Autodesk Fusion 360 part; units mm, degrees
(part 13 of 18)
  line L7813 (180.127, -19.7823) -> (179.311, -19.7823)
  line L7814 (179.311, -19.5783) -> (180.127, -19.5783)
  line L7815 (180.127, -19.5783) -> (180.127, -19.7823)
  line L7816 (176.8331, -76.9578) -> (177.6491, -76.9578)
  line L7817 (177.6491, -76.9578) -> (177.6491, -76.7538)
  line L7818 (177.6491, -76.7538) -> (176.8331, -76.7538)
  line L7819 (176.8331, -76.7538) -> (176.8331, -76.9578)
  line L7820 (179.821, -77.5359) -> (179.617, -77.5359)
  line L7821 (179.617, -76.1758) -> (179.821, -76.1758)
  line L7822 (179.617, -77.5359) -> (179.617, -76.1758)
  line L7823 (179.821, -76.1758) -> (179.821, -77.5359)
  line L7824 (179.311, -76.9579) -> (179.311, -76.7538)
  line L7825 (179.311, -76.7538) -> (180.127, -76.7538)
  line L7826 (180.127, -76.7538) -> (180.127, -76.9579)
  line L7827 (180.127, -76.9579) -> (179.311, -76.9579)
  line L7828 (176.8331, -57.6911) -> (176.8331, -57.8951)
  line L7829 (176.8331, -57.8951) -> (177.6491, -57.8951)
  line L7830 (177.6491, -57.8951) -> (177.6491, -57.6911)
  line L7831 (177.6491, -57.6911) -> (176.8331, -57.6911)
  line L7832 (179.617, -58.4731) -> (179.617, -57.1131)
  line L7833 (179.821, -57.1131) -> (179.821, -58.4731)
  line L7834 (179.821, -58.4731) -> (179.617, -58.4731)
  line L7835 (179.617, -57.1131) -> (179.821, -57.1131)
  line L7836 (180.127, -57.8951) -> (179.311, -57.8951)
  line L7837 (179.311, -57.6911) -> (180.127, -57.6911)
  line L7838 (180.127, -57.6911) -> (180.127, -57.8951)
  line L7839 (179.311, -57.8951) -> (179.311, -57.6911)
  line L7840 (176.8331, -38.6283) -> (176.8331, -38.8324)
  line L7841 (176.8331, -38.8324) -> (177.6491, -38.8324)
  line L7842 (177.6491, -38.6283) -> (176.8331, -38.6283)
  line L7843 (177.6491, -38.8324) -> (177.6491, -38.6283)
  line L7844 (179.617, -38.0504) -> (179.821, -38.0504)
  line L7845 (179.821, -39.4104) -> (179.617, -39.4104)
  line L7846 (179.821, -38.0504) -> (179.821, -39.4104)
  line L7847 (179.617, -39.4104) -> (179.617, -38.0504)
  line L7848 (179.311, -38.6284) -> (180.127, -38.6284)
  line L7849 (180.127, -38.6284) -> (180.127, -38.8324)
  line L7850 (180.127, -38.8324) -> (179.311, -38.8324)
  line L7851 (179.311, -38.8324) -> (179.311, -38.6284)
  line L7852 (100.6329, -76.7538) -> (100.6329, -76.9578)
  line L7853 (101.4489, -76.7538) -> (100.6329, -76.7538)
  line L7854 (100.6329, -76.9578) -> (101.4489, -76.9578)
  line L7855 (101.4489, -76.9578) -> (101.4489, -76.7538)
  line L7856 (103.4168, -76.1758) -> (103.6208, -76.1758)
  line L7857 (103.6208, -77.5359) -> (103.4168, -77.5359)
  line L7858 (103.6208, -76.1758) -> (103.6208, -77.5359)
  line L7859 (103.4168, -77.5359) -> (103.4168, -76.1758)
  line L7860 (103.9268, -76.9579) -> (103.1108, -76.9579)
  line L7861 (103.1108, -76.7538) -> (103.9268, -76.7538)
  line L7862 (103.9268, -76.7538) -> (103.9268, -76.9579)
  line L7863 (103.1108, -76.9579) -> (103.1108, -76.7538)
  line L7864 (101.4489, -57.6911) -> (100.6329, -57.6911)
  line L7865 (101.4489, -57.8951) -> (101.4489, -57.6911)
  line L7866 (100.6329, -57.6911) -> (100.6329, -57.8951)
  line L7867 (100.6329, -57.8951) -> (101.4489, -57.8951)
  line L7868 (103.4168, -58.4731) -> (103.4168, -57.1131)
  line L7869 (103.4168, -57.1131) -> (103.6208, -57.1131)
  line L7870 (103.6208, -58.4731) -> (103.4168, -58.4731)
  line L7871 (103.6208, -57.1131) -> (103.6208, -58.4731)
  line L7872 (103.9268, -57.8951) -> (103.1108, -57.8951)
  line L7873 (103.9268, -57.6911) -> (103.9268, -57.8951)
  line L7874 (103.1108, -57.6911) -> (103.9268, -57.6911)
  line L7875 (103.1108, -57.8951) -> (103.1108, -57.6911)
  line L7876 (101.4489, -19.5783) -> (100.6329, -19.5783)
  line L7877 (100.6329, -19.5783) -> (100.6329, -19.7823)
  line L7878 (101.4489, -19.7823) -> (101.4489, -19.5783)
  line L7879 (100.6329, -19.7823) -> (101.4489, -19.7823)
  line L7880 (103.6208, -20.3604) -> (103.4168, -20.3604)
  line L7881 (103.6208, -19.0003) -> (103.6208, -20.3604)
  line L7882 (103.4168, -19.0003) -> (103.6208, -19.0003)
  line L7883 (103.4168, -20.3604) -> (103.4168, -19.0003)
  line L7884 (103.1108, -19.7823) -> (103.1108, -19.5783)
  line L7885 (103.9268, -19.7823) -> (103.1108, -19.7823)
  line L7886 (103.9268, -19.5783) -> (103.9268, -19.7823)
  line L7887 (103.1108, -19.5783) -> (103.9268, -19.5783)
  line L7888 (100.6329, -38.8324) -> (101.4489, -38.8324)
  line L7889 (101.4489, -38.6283) -> (100.6329, -38.6283)
  line L7890 (101.4489, -38.8324) -> (101.4489, -38.6283)
  line L7891 (100.6329, -38.6283) -> (100.6329, -38.8324)
  line L7892 (103.4168, -39.4104) -> (103.4168, -38.0504)
  line L7893 (103.6208, -38.0504) -> (103.6208, -39.4104)
  line L7894 (103.6208, -39.4104) -> (103.4168, -39.4104)
  line L7895 (103.4168, -38.0504) -> (103.6208, -38.0504)
  line L7896 (103.1108, -38.8324) -> (103.1108, -38.6284)
  line L7897 (103.9268, -38.8324) -> (103.1108, -38.8324)
  line L7898 (103.9268, -38.6284) -> (103.9268, -38.8324)
  line L7899 (103.1108, -38.6284) -> (103.9268, -38.6284)
  line L7900 (120.499, -19.5783) -> (119.683, -19.5783)
  line L7901 (119.683, -19.5783) -> (119.683, -19.7823)
  line L7902 (120.499, -19.7823) -> (120.499, -19.5783)
  line L7903 (119.683, -19.7823) -> (120.499, -19.7823)
  line L7904 (122.6709, -19.0003) -> (122.6709, -20.3604)
  line L7905 (122.4669, -20.3604) -> (122.4669, -19.0003)
  line L7906 (122.4669, -19.0003) -> (122.6709, -19.0003)
  line L7907 (122.6709, -20.3604) -> (122.4669, -20.3604)
  line L7908 (122.1609, -19.7823) -> (122.1609, -19.5783)
  line L7909 (122.1609, -19.5783) -> (122.9769, -19.5783)
  line L7910 (122.9769, -19.7823) -> (122.1609, -19.7823)
  line L7911 (122.9769, -19.5783) -> (122.9769, -19.7823)
  line L7912 (119.683, -57.8951) -> (120.499, -57.8951)
  line L7913 (120.499, -57.8951) -> (120.499, -57.6911)
  line L7914 (119.683, -57.6911) -> (119.683, -57.8951)
  line L7915 (120.499, -57.6911) -> (119.683, -57.6911)
  line L7916 (122.4669, -57.1131) -> (122.6709, -57.1131)
  line L7917 (122.6709, -57.1131) -> (122.6709, -58.4731)
  line L7918 (122.6709, -58.4731) -> (122.4669, -58.4731)
  line L7919 (122.4669, -58.4731) -> (122.4669, -57.1131)
  line L7920 (122.9769, -57.8951) -> (122.1609, -57.8951)
  line L7921 (122.1609, -57.8951) -> (122.1609, -57.6911)
  line L7922 (122.9769, -57.6911) -> (122.9769, -57.8951)
  line L7923 (122.1609, -57.6911) -> (122.9769, -57.6911)
  line L7924 (119.683, -38.6283) -> (119.683, -38.8324)
  line L7925 (119.683, -38.8324) -> (120.499, -38.8324)
  line L7926 (120.499, -38.6283) -> (119.683, -38.6283)
  line L7927 (120.499, -38.8324) -> (120.499, -38.6283)
  line L7928 (122.6709, -38.0504) -> (122.6709, -39.4104)
  line L7929 (122.6709, -39.4104) -> (122.4669, -39.4104)
  line L7930 (122.4669, -38.0504) -> (122.6709, -38.0504)
  line L7931 (122.4669, -39.4104) -> (122.4669, -38.0504)
  line L7932 (122.9769, -38.8324) -> (122.1609, -38.8324)
  line L7933 (122.1609, -38.6284) -> (122.9769, -38.6284)
  line L7934 (122.1609, -38.8324) -> (122.1609, -38.6284)
  line L7935 (122.9769, -38.6284) -> (122.9769, -38.8324)
  line L7936 (120.499, -76.9578) -> (120.499, -76.7538)
  line L7937 (120.499, -76.7538) -> (119.683, -76.7538)
  line L7938 (119.683, -76.7538) -> (119.683, -76.9578)
  line L7939 (119.683, -76.9578) -> (120.499, -76.9578)
  line L7940 (122.4669, -76.1758) -> (122.6709, -76.1758)
  line L7941 (122.6709, -76.1758) -> (122.6709, -77.5359)
  line L7942 (122.4669, -77.5359) -> (122.4669, -76.1758)
  line L7943 (122.6709, -77.5359) -> (122.4669, -77.5359)
  line L7944 (122.1609, -76.9579) -> (122.1609, -76.7538)
  line L7945 (122.9769, -76.7538) -> (122.9769, -76.9579)
  line L7946 (122.1609, -76.7538) -> (122.9769, -76.7538)
  line L7947 (122.9769, -76.9579) -> (122.1609, -76.9579)
  line L7948 (6.1988, -76.7538) -> (5.3828, -76.7538)
  line L7949 (5.3828, -76.9578) -> (6.1988, -76.9578)
  line L7950 (6.1988, -76.9578) -> (6.1988, -76.7538)
  line L7951 (5.3828, -76.7538) -> (5.3828, -76.9578)
  line L7952 (8.1666, -77.5359) -> (8.1666, -76.1758)
  line L7953 (8.1666, -76.1758) -> (8.3706, -76.1758)
  line L7954 (8.3706, -77.5359) -> (8.1666, -77.5359)
  line L7955 (8.3706, -76.1758) -> (8.3706, -77.5359)
  line L7956 (8.6766, -76.9579) -> (7.8606, -76.9579)
  line L7957 (7.8606, -76.7538) -> (8.6766, -76.7538)
  line L7958 (8.6766, -76.7538) -> (8.6766, -76.9579)
  line L7959 (7.8606, -76.9579) -> (7.8606, -76.7538)
  line L7960 (24.4328, -76.9578) -> (25.2488, -76.9578)
  line L7961 (25.2488, -76.7538) -> (24.4328, -76.7538)
  line L7962 (25.2488, -76.9578) -> (25.2488, -76.7538)
  line L7963 (24.4328, -76.7538) -> (24.4328, -76.9578)
  line L7964 (27.2167, -77.5359) -> (27.2167, -76.1758)
  line L7965 (27.2167, -76.1758) -> (27.4207, -76.1758)
  line L7966 (27.4207, -77.5359) -> (27.2167, -77.5359)
  line L7967 (27.4207, -76.1758) -> (27.4207, -77.5359)
  line L7968 (26.9107, -76.9579) -> (26.9107, -76.7538)
  line L7969 (27.7267, -76.7538) -> (27.7267, -76.9579)
  line L7970 (27.7267, -76.9579) -> (26.9107, -76.9579)
  line L7971 (26.9107, -76.7538) -> (27.7267, -76.7538)
  line L7972 (43.4828, -76.7538) -> (43.4828, -76.9578)
  line L7973 (44.2988, -76.9578) -> (44.2988, -76.7538)
  line L7974 (43.4828, -76.9578) -> (44.2988, -76.9578)
  line L7975 (44.2988, -76.7538) -> (43.4828, -76.7538)
  line L7976 (46.2667, -77.5359) -> (46.2667, -76.1758)
  line L7977 (46.4707, -76.1758) -> (46.4707, -77.5359)
  line L7978 (46.4707, -77.5359) -> (46.2667, -77.5359)
  line L7979 (46.2667, -76.1758) -> (46.4707, -76.1758)
  line L7980 (45.9607, -76.7538) -> (46.7767, -76.7538)
  line L7981 (45.9607, -76.9579) -> (45.9607, -76.7538)
  line L7982 (46.7767, -76.9579) -> (45.9607, -76.9579)
  line L7983 (46.7767, -76.7538) -> (46.7767, -76.9579)
  line L7984 (62.5329, -19.5783) -> (62.5329, -19.7823)
  line L7985 (62.5329, -19.7823) -> (63.3489, -19.7823)
  line L7986 (63.3489, -19.5783) -> (62.5329, -19.5783)
  line L7987 (63.3489, -19.7823) -> (63.3489, -19.5783)
  line L7988 (65.3167, -20.3604) -> (65.3167, -19.0003)
  line L7989 (65.5208, -19.0003) -> (65.5208, -20.3604)
  line L7990 (65.5208, -20.3604) -> (65.3167, -20.3604)
  line L7991 (65.3167, -19.0003) -> (65.5208, -19.0003)
  line L7992 (65.8267, -19.7823) -> (65.0107, -19.7823)
  line L7993 (65.8267, -19.5783) -> (65.8267, -19.7823)
  line L7994 (65.0107, -19.5783) -> (65.8267, -19.5783)
  line L7995 (65.0107, -19.7823) -> (65.0107, -19.5783)
  line L7996 (62.5329, -76.7538) -> (62.5329, -76.9578)
  line L7997 (62.5329, -76.9578) -> (63.3489, -76.9578)
  line L7998 (63.3489, -76.9578) -> (63.3489, -76.7538)
  line L7999 (63.3489, -76.7538) -> (62.5329, -76.7538)
  line L8000 (65.5208, -77.5359) -> (65.3167, -77.5359)
  line L8001 (65.5208, -76.1758) -> (65.5208, -77.5359)
  line L8002 (65.3167, -77.5359) -> (65.3167, -76.1758)
  line L8003 (65.3167, -76.1758) -> (65.5208, -76.1758)
  line L8004 (65.0107, -76.9579) -> (65.0107, -76.7538)
  line L8005 (65.8267, -76.7538) -> (65.8267, -76.9579)
  line L8006 (65.8267, -76.9579) -> (65.0107, -76.9579)
  line L8007 (65.0107, -76.7538) -> (65.8267, -76.7538)
  line L8008 (63.3489, -38.8324) -> (63.3489, -38.6283)
  line L8009 (62.5329, -38.6283) -> (62.5329, -38.8324)
  line L8010 (62.5329, -38.8324) -> (63.3489, -38.8324)
  line L8011 (63.3489, -38.6283) -> (62.5329, -38.6283)
  line L8012 (65.3167, -38.0504) -> (65.5208, -38.0504)
  line L8013 (65.5208, -38.0504) -> (65.5208, -39.4104)
  line L8014 (65.3167, -39.4104) -> (65.3167, -38.0504)
  line L8015 (65.5208, -39.4104) -> (65.3167, -39.4104)
  line L8016 (65.0107, -38.6284) -> (65.8267, -38.6284)
  line L8017 (65.8267, -38.6284) -> (65.8267, -38.8324)
  line L8018 (65.8267, -38.8324) -> (65.0107, -38.8324)
  line L8019 (65.0107, -38.8324) -> (65.0107, -38.6284)
  line L8020 (62.5329, -57.6911) -> (62.5329, -57.8951)
  line L8021 (62.5329, -57.8951) -> (63.3489, -57.8951)
  line L8022 (63.3489, -57.6911) -> (62.5329, -57.6911)
  line L8023 (63.3489, -57.8951) -> (63.3489, -57.6911)
  line L8024 (65.3167, -57.1131) -> (65.5208, -57.1131)
  line L8025 (65.5208, -58.4731) -> (65.3167, -58.4731)
  line L8026 (65.3167, -58.4731) -> (65.3167, -57.1131)
  line L8027 (65.5208, -57.1131) -> (65.5208, -58.4731)
  line L8028 (65.8267, -57.6911) -> (65.8267, -57.8951)
  line L8029 (65.8267, -57.8951) -> (65.0107, -57.8951)
  line L8030 (65.0107, -57.6911) -> (65.8267, -57.6911)
  line L8031 (65.0107, -57.8951) -> (65.0107, -57.6911)
  line L8032 (82.3989, -38.6283) -> (81.5829, -38.6283)
  line L8033 (81.5829, -38.6283) -> (81.5829, -38.8324)
  line L8034 (82.3989, -38.8324) -> (82.3989, -38.6283)
  line L8035 (81.5829, -38.8324) -> (82.3989, -38.8324)
  line L8036 (84.5708, -38.0504) -> (84.5708, -39.4104)
  line L8037 (84.5708, -39.4104) -> (84.3668, -39.4104)
  line L8038 (84.3668, -39.4104) -> (84.3668, -38.0504)
  line L8039 (84.3668, -38.0504) -> (84.5708, -38.0504)
  line L8040 (84.0608, -38.8324) -> (84.0608, -38.6284)
  line L8041 (84.0608, -38.6284) -> (84.8768, -38.6284)
  line L8042 (84.8768, -38.6284) -> (84.8768, -38.8324)
  line L8043 (84.8768, -38.8324) -> (84.0608, -38.8324)
  line L8044 (82.3989, -76.7538) -> (81.5829, -76.7538)
  line L8045 (81.5829, -76.7538) -> (81.5829, -76.9578)
  line L8046 (81.5829, -76.9578) -> (82.3989, -76.9578)
  line L8047 (82.3989, -76.9578) -> (82.3989, -76.7538)
  line L8048 (84.3668, -77.5359) -> (84.3668, -76.1758)
  line L8049 (84.5708, -77.5359) -> (84.3668, -77.5359)
  line L8050 (84.3668, -76.1758) -> (84.5708, -76.1758)
  line L8051 (84.5708, -76.1758) -> (84.5708, -77.5359)
  line L8052 (84.0608, -76.7538) -> (84.8768, -76.7538)
  line L8053 (84.0608, -76.9579) -> (84.0608, -76.7538)
  line L8054 (84.8768, -76.7538) -> (84.8768, -76.9579)
  line L8055 (84.8768, -76.9579) -> (84.0608, -76.9579)
  line L8056 (81.5829, -19.5783) -> (81.5829, -19.7823)
  line L8057 (82.3989, -19.7823) -> (82.3989, -19.5783)
  line L8058 (81.5829, -19.7823) -> (82.3989, -19.7823)
  line L8059 (82.3989, -19.5783) -> (81.5829, -19.5783)
  line L8060 (84.3668, -19.0003) -> (84.5708, -19.0003)
  line L8061 (84.5708, -19.0003) -> (84.5708, -20.3604)
  line L8062 (84.5708, -20.3604) -> (84.3668, -20.3604)
  line L8063 (84.3668, -20.3604) -> (84.3668, -19.0003)
  line L8064 (84.0608, -19.7823) -> (84.0608, -19.5783)
  line L8065 (84.8768, -19.7823) -> (84.0608, -19.7823)
  line L8066 (84.0608, -19.5783) -> (84.8768, -19.5783)
  line L8067 (84.8768, -19.5783) -> (84.8768, -19.7823)
  line L8068 (82.3989, -57.8951) -> (82.3989, -57.6911)
  line L8069 (81.5829, -57.6911) -> (81.5829, -57.8951)
  line L8070 (81.5829, -57.8951) -> (82.3989, -57.8951)
  line L8071 (82.3989, -57.6911) -> (81.5829, -57.6911)
  line L8072 (84.5708, -57.1131) -> (84.5708, -58.4731)
  line L8073 (84.5708, -58.4731) -> (84.3668, -58.4731)
  line L8074 (84.3668, -57.1131) -> (84.5708, -57.1131)
  line L8075 (84.3668, -58.4731) -> (84.3668, -57.1131)
  line L8076 (84.8768, -57.8951) -> (84.0608, -57.8951)
  line L8077 (84.0608, -57.6911) -> (84.8768, -57.6911)
  line L8078 (84.8768, -57.6911) -> (84.8768, -57.8951)
  line L8079 (84.0608, -57.8951) -> (84.0608, -57.6911)
  line L8080 (6.1988, -57.8951) -> (6.1988, -57.6911)
  line L8081 (5.3828, -57.6911) -> (5.3828, -57.8951)
  line L8082 (5.3828, -57.8951) -> (6.1988, -57.8951)
  line L8083 (6.1988, -57.6911) -> (5.3828, -57.6911)
  line L8084 (8.1666, -58.4731) -> (8.1666, -57.1131)
  line L8085 (8.3706, -58.4731) -> (8.1666, -58.4731)
  line L8086 (8.1666, -57.1131) -> (8.3706, -57.1131)
  line L8087 (8.3706, -57.1131) -> (8.3706, -58.4731)
  line L8088 (7.8606, -57.6911) -> (8.6766, -57.6911)
  line L8089 (8.6766, -57.8951) -> (7.8606, -57.8951)
  line L8090 (8.6766, -57.6911) -> (8.6766, -57.8951)
  line L8091 (7.8606, -57.8951) -> (7.8606, -57.6911)
  line L8092 (5.3828, -19.5783) -> (5.3828, -19.7823)
  line L8093 (5.3828, -19.7823) -> (6.1988, -19.7823)
  line L8094 (6.1988, -19.5783) -> (5.3828, -19.5783)
  line L8095 (6.1988, -19.7823) -> (6.1988, -19.5783)
  line L8096 (8.3706, -20.3604) -> (8.1666, -20.3604)
  line L8097 (8.1666, -20.3604) -> (8.1666, -19.0003)
  line L8098 (8.1666, -19.0003) -> (8.3706, -19.0003)
  line L8099 (8.3706, -19.0003) -> (8.3706, -20.3604)
  line L8100 (7.8606, -19.7823) -> (7.8606, -19.5783)
  line L8101 (8.6766, -19.7823) -> (7.8606, -19.7823)
  line L8102 (7.8606, -19.5783) -> (8.6766, -19.5783)
  line L8103 (8.6766, -19.5783) -> (8.6766, -19.7823)
  line L8104 (6.1988, -38.8324) -> (6.1988, -38.6283)
  line L8105 (5.3828, -38.6283) -> (5.3828, -38.8324)
  line L8106 (6.1988, -38.6283) -> (5.3828, -38.6283)
  line L8107 (5.3828, -38.8324) -> (6.1988, -38.8324)
  line L8108 (8.1666, -39.4104) -> (8.1666, -38.0504)
  line L8109 (8.1666, -38.0504) -> (8.3706, -38.0504)
  line L8110 (8.3706, -39.4104) -> (8.1666, -39.4104)
  line L8111 (8.3706, -38.0504) -> (8.3706, -39.4104)
  line L8112 (7.8606, -38.8324) -> (7.8606, -38.6284)
  line L8113 (7.8606, -38.6284) -> (8.6766, -38.6284)
  line L8114 (8.6766, -38.6284) -> (8.6766, -38.8324)
  line L8115 (8.6766, -38.8324) -> (7.8606, -38.8324)
  line L8116 (25.2488, -38.8324) -> (25.2488, -38.6283)
  line L8117 (24.4328, -38.6283) -> (24.4328, -38.8324)
  line L8118 (25.2488, -38.6283) -> (24.4328, -38.6283)
  line L8119 (24.4328, -38.8324) -> (25.2488, -38.8324)
  line L8120 (27.2167, -39.4104) -> (27.2167, -38.0504)
  line L8121 (27.4207, -39.4104) -> (27.2167, -39.4104)
  line L8122 (27.2167, -38.0504) -> (27.4207, -38.0504)
  line L8123 (27.4207, -38.0504) -> (27.4207, -39.4104)
  line L8124 (26.9107, -38.8324) -> (26.9107, -38.6284)
  line L8125 (27.7267, -38.8324) -> (26.9107, -38.8324)
  line L8126 (27.7267, -38.6284) -> (27.7267, -38.8324)
  line L8127 (26.9107, -38.6284) -> (27.7267, -38.6284)
  line L8128 (24.4328, -19.7823) -> (25.2488, -19.7823)
  line L8129 (25.2488, -19.5783) -> (24.4328, -19.5783)
  line L8130 (25.2488, -19.7823) -> (25.2488, -19.5783)
  line L8131 (24.4328, -19.5783) -> (24.4328, -19.7823)
  line L8132 (27.2167, -20.3604) -> (27.2167, -19.0003)
  line L8133 (27.4207, -20.3604) -> (27.2167, -20.3604)
  line L8134 (27.4207, -19.0003) -> (27.4207, -20.3604)
  line L8135 (27.2167, -19.0003) -> (27.4207, -19.0003)
  line L8136 (27.7267, -19.7823) -> (26.9107, -19.7823)
  line L8137 (26.9107, -19.5783) -> (27.7267, -19.5783)
  line L8138 (27.7267, -19.5783) -> (27.7267, -19.7823)
  line L8139 (26.9107, -19.7823) -> (26.9107, -19.5783)
  line L8140 (25.2488, -57.6911) -> (24.4328, -57.6911)
  line L8141 (24.4328, -57.8951) -> (25.2488, -57.8951)
  line L8142 (24.4328, -57.6911) -> (24.4328, -57.8951)
  line L8143 (25.2488, -57.8951) -> (25.2488, -57.6911)
  line L8144 (27.4207, -58.4731) -> (27.2167, -58.4731)
  line L8145 (27.4207, -57.1131) -> (27.4207, -58.4731)
  line L8146 (27.2167, -57.1131) -> (27.4207, -57.1131)
  line L8147 (27.2167, -58.4731) -> (27.2167, -57.1131)
  line L8148 (27.7267, -57.8951) -> (26.9107, -57.8951)
  line L8149 (26.9107, -57.6911) -> (27.7267, -57.6911)
  line L8150 (27.7267, -57.6911) -> (27.7267, -57.8951)
  line L8151 (26.9107, -57.8951) -> (26.9107, -57.6911)
  line L8152 (43.4828, -19.7823) -> (44.2988, -19.7823)
  line L8153 (43.4828, -19.5783) -> (43.4828, -19.7823)
  line L8154 (44.2988, -19.7823) -> (44.2988, -19.5783)
  line L8155 (44.2988, -19.5783) -> (43.4828, -19.5783)
  line L8156 (46.4707, -20.3604) -> (46.2667, -20.3604)
  line L8157 (46.2667, -20.3604) -> (46.2667, -19.0003)
  line L8158 (46.4707, -19.0003) -> (46.4707, -20.3604)
  line L8159 (46.2667, -19.0003) -> (46.4707, -19.0003)
  line L8160 (45.9607, -19.7823) -> (45.9607, -19.5783)
  line L8161 (46.7767, -19.5783) -> (46.7767, -19.7823)
  line L8162 (45.9607, -19.5783) -> (46.7767, -19.5783)
  line L8163 (46.7767, -19.7823) -> (45.9607, -19.7823)
  line L8164 (43.4828, -57.8951) -> (44.2988, -57.8951)
  line L8165 (44.2988, -57.6911) -> (43.4828, -57.6911)
  line L8166 (44.2988, -57.8951) -> (44.2988, -57.6911)
  line L8167 (43.4828, -57.6911) -> (43.4828, -57.8951)
  line L8168 (46.4707, -58.4731) -> (46.2667, -58.4731)
  line L8169 (46.4707, -57.1131) -> (46.4707, -58.4731)
  line L8170 (46.2667, -58.4731) -> (46.2667, -57.1131)
  line L8171 (46.2667, -57.1131) -> (46.4707, -57.1131)
  line L8172 (45.9607, -57.8951) -> (45.9607, -57.6911)
  line L8173 (45.9607, -57.6911) -> (46.7767, -57.6911)
  line L8174 (46.7767, -57.8951) -> (45.9607, -57.8951)
  line L8175 (46.7767, -57.6911) -> (46.7767, -57.8951)
  line L8176 (44.2988, -38.8324) -> (44.2988, -38.6283)
  line L8177 (43.4828, -38.8324) -> (44.2988, -38.8324)
  line L8178 (43.4828, -38.6283) -> (43.4828, -38.8324)
  line L8179 (44.2988, -38.6283) -> (43.4828, -38.6283)
  line L8180 (46.4707, -39.4104) -> (46.2667, -39.4104)
  line L8181 (46.2667, -38.0504) -> (46.4707, -38.0504)
  line L8182 (46.4707, -38.0504) -> (46.4707, -39.4104)
  line L8183 (46.2667, -39.4104) -> (46.2667, -38.0504)
  line L8184 (46.7767, -38.6284) -> (46.7767, -38.8324)
  line L8185 (45.9607, -38.6284) -> (46.7767, -38.6284)
  line L8186 (46.7767, -38.8324) -> (45.9607, -38.8324)
  line L8187 (45.9607, -38.8324) -> (45.9607, -38.6284)
  line L8188 (215.7492, -19.5783) -> (214.9332, -19.5783)
  line L8189 (214.9332, -19.7823) -> (215.7492, -19.7823)
  line L8190 (215.7492, -19.7823) -> (215.7492, -19.5783)
  line L8191 (214.9332, -19.5783) -> (214.9332, -19.7823)
  line L8192 (217.717, -19.0003) -> (217.9211, -19.0003)
  line L8193 (217.9211, -20.3604) -> (217.717, -20.3604)
  line L8194 (217.717, -20.3604) -> (217.717, -19.0003)
  line L8195 (217.9211, -19.0003) -> (217.9211, -20.3604)
  line L8196 (217.411, -19.5783) -> (218.2271, -19.5783)
  line L8197 (218.2271, -19.5783) -> (218.2271, -19.7823)
  line L8198 (218.2271, -19.7823) -> (217.411, -19.7823)
  line L8199 (217.411, -19.7823) -> (217.411, -19.5783)
  line L8200 (214.9332, -76.9578) -> (215.7492, -76.9578)
  line L8201 (215.7492, -76.9578) -> (215.7492, -76.7538)
  line L8202 (214.9332, -76.7538) -> (214.9332, -76.9578)
  line L8203 (215.7492, -76.7538) -> (214.9332, -76.7538)
  line L8204 (217.9211, -76.1758) -> (217.9211, -77.5359)
  line L8205 (217.717, -76.1758) -> (217.9211, -76.1758)
  line L8206 (217.717, -77.5359) -> (217.717, -76.1758)
  line L8207 (217.9211, -77.5359) -> (217.717, -77.5359)
  line L8208 (218.2271, -76.7538) -> (218.2271, -76.9579)
  line L8209 (218.2271, -76.9579) -> (217.411, -76.9579)
  line L8210 (217.411, -76.7538) -> (218.2271, -76.7538)
  line L8211 (217.411, -76.9579) -> (217.411, -76.7538)
  line L8212 (215.7492, -57.6911) -> (214.9332, -57.6911)
  line L8213 (215.7492, -57.8951) -> (215.7492, -57.6911)
  line L8214 (214.9332, -57.6911) -> (214.9332, -57.8951)
  line L8215 (214.9332, -57.8951) -> (215.7492, -57.8951)
  line L8216 (217.9211, -57.1131) -> (217.9211, -58.4731)
  line L8217 (217.717, -58.4731) -> (217.717, -57.1131)
  line L8218 (217.9211, -58.4731) -> (217.717, -58.4731)
  line L8219 (217.717, -57.1131) -> (217.9211, -57.1131)
  line L8220 (217.411, -57.8951) -> (217.411, -57.6911)
  line L8221 (217.411, -57.6911) -> (218.2271, -57.6911)
  line L8222 (218.2271, -57.6911) -> (218.2271, -57.8951)
  line L8223 (218.2271, -57.8951) -> (217.411, -57.8951)
  line L8224 (215.7492, -38.8324) -> (215.7492, -38.6283)
  line L8225 (214.9332, -38.6283) -> (214.9332, -38.8324)
  line L8226 (215.7492, -38.6283) -> (214.9332, -38.6283)
  line L8227 (214.9332, -38.8324) -> (215.7492, -38.8324)
  line L8228 (217.717, -38.0504) -> (217.9211, -38.0504)
  line L8229 (217.717, -39.4104) -> (217.717, -38.0504)
  line L8230 (217.9211, -38.0504) -> (217.9211, -39.4104)
  line L8231 (217.9211, -39.4104) -> (217.717, -39.4104)
  line L8232 (217.411, -38.6284) -> (218.2271, -38.6284)
  line L8233 (218.2271, -38.6284) -> (218.2271, -38.8324)
  line L8234 (217.411, -38.8324) -> (217.411, -38.6284)
  line L8235 (218.2271, -38.8324) -> (217.411, -38.8324)
  line L8236 (196.6991, -38.8324) -> (196.6991, -38.6283)
  line L8237 (195.8831, -38.6283) -> (195.8831, -38.8324)
  line L8238 (196.6991, -38.6283) -> (195.8831, -38.6283)
  line L8239 (195.8831, -38.8324) -> (196.6991, -38.8324)
  line L8240 (198.871, -39.4104) -> (198.667, -39.4104)
  line L8241 (198.667, -39.4104) -> (198.667, -38.0504)
  line L8242 (198.667, -38.0504) -> (198.871, -38.0504)
  line L8243 (198.871, -38.0504) -> (198.871, -39.4104)
  line L8244 (198.361, -38.6284) -> (199.177, -38.6284)
  line L8245 (199.177, -38.8324) -> (198.361, -38.8324)
  line L8246 (199.177, -38.6284) -> (199.177, -38.8324)
  line L8247 (198.361, -38.8324) -> (198.361, -38.6284)
  line L8248 (195.8831, -76.7538) -> (195.8831, -76.9578)
  line L8249 (196.6991, -76.9578) -> (196.6991, -76.7538)
  line L8250 (195.8831, -76.9578) -> (196.6991, -76.9578)
  line L8251 (196.6991, -76.7538) -> (195.8831, -76.7538)
  line L8252 (198.667, -77.5359) -> (198.667, -76.1758)
  line L8253 (198.871, -77.5359) -> (198.667, -77.5359)
  line L8254 (198.871, -76.1758) -> (198.871, -77.5359)
  line L8255 (198.667, -76.1758) -> (198.871, -76.1758)
  line L8256 (199.177, -76.9579) -> (198.361, -76.9579)
  line L8257 (198.361, -76.7538) -> (199.177, -76.7538)
  line L8258 (199.177, -76.7538) -> (199.177, -76.9579)
  line L8259 (198.361, -76.9579) -> (198.361, -76.7538)
  line L8260 (196.6991, -57.8951) -> (196.6991, -57.6911)
  line L8261 (195.8831, -57.8951) -> (196.6991, -57.8951)
  line L8262 (195.8831, -57.6911) -> (195.8831, -57.8951)
  line L8263 (196.6991, -57.6911) -> (195.8831, -57.6911)
  line L8264 (198.667, -57.1131) -> (198.871, -57.1131)
  line L8265 (198.871, -57.1131) -> (198.871, -58.4731)
  line L8266 (198.871, -58.4731) -> (198.667, -58.4731)
  line L8267 (198.667, -58.4731) -> (198.667, -57.1131)
  line L8268 (199.177, -57.8951) -> (198.361, -57.8951)
  line L8269 (198.361, -57.8951) -> (198.361, -57.6911)
  line L8270 (199.177, -57.6911) -> (199.177, -57.8951)
  line L8271 (198.361, -57.6911) -> (199.177, -57.6911)
  line L8272 (195.8831, -19.7823) -> (196.6991, -19.7823)
  line L8273 (196.6991, -19.7823) -> (196.6991, -19.5783)
  line L8274 (196.6991, -19.5783) -> (195.8831, -19.5783)
  line L8275 (195.8831, -19.5783) -> (195.8831, -19.7823)
  line L8276 (198.667, -19.0003) -> (198.871, -19.0003)
  line L8277 (198.871, -19.0003) -> (198.871, -20.3604)
  line L8278 (198.667, -20.3604) -> (198.667, -19.0003)
  line L8279 (198.871, -20.3604) -> (198.667, -20.3604)
  line L8280 (198.361, -19.7823) -> (198.361, -19.5783)
  line L8281 (199.177, -19.7823) -> (198.361, -19.7823)
  line L8282 (198.361, -19.5783) -> (199.177, -19.5783)
  line L8283 (199.177, -19.5783) -> (199.177, -19.7823)
  arc A1890 (207.1995, -6.1629) -> (207.3494, -6.1629) centre (207.2744, -6.1629) ccw
  arc A1891 (207.3494, -6.1629) -> (207.1995, -6.1629) centre (207.2744, -6.1629) ccw
  arc A1892 (212.8031, -3.2765) -> (213.0033, -3.2765) centre (212.9032, -3.2765) ccw
  arc A1893 (213.0033, -3.2765) -> (212.8031, -3.2765) centre (212.9032, -3.2765) ccw
  line L8284 (139.549, -76.7538) -> (138.733, -76.7538)
  line L8285 (138.733, -76.7538) -> (138.733, -76.9578)
  line L8286 (139.549, -76.9578) -> (139.549, -76.7538)
  line L8287 (138.733, -76.9578) -> (139.549, -76.9578)
  line L8288 (141.7209, -76.1758) -> (141.7209, -77.5359)
  line L8289 (141.5169, -77.5359) -> (141.5169, -76.1758)
  line L8290 (141.5169, -76.1758) -> (141.7209, -76.1758)
  line L8291 (141.7209, -77.5359) -> (141.5169, -77.5359)
  line L8292 (141.2109, -76.7538) -> (142.0269, -76.7538)
  line L8293 (142.0269, -76.9579) -> (141.2109, -76.9579)
  line L8294 (142.0269, -76.7538) -> (142.0269, -76.9579)
  line L8295 (141.2109, -76.9579) -> (141.2109, -76.7538)
  line L8296 (139.549, -19.5783) -> (138.733, -19.5783)
  line L8297 (138.733, -19.7823) -> (139.549, -19.7823)
  line L8298 (138.733, -19.5783) -> (138.733, -19.7823)
  line L8299 (139.549, -19.7823) -> (139.549, -19.5783)
  line L8300 (141.5169, -20.3604) -> (141.5169, -19.0003)
  line L8301 (141.5169, -19.0003) -> (141.7209, -19.0003)
  line L8302 (141.7209, -19.0003) -> (141.7209, -20.3604)
  line L8303 (141.7209, -20.3604) -> (141.5169, -20.3604)
  line L8304 (141.2109, -19.5783) -> (142.0269, -19.5783)
  line L8305 (141.2109, -19.7823) -> (141.2109, -19.5783)
  line L8306 (142.0269, -19.5783) -> (142.0269, -19.7823)
  line L8307 (142.0269, -19.7823) -> (141.2109, -19.7823)
  line L8308 (138.733, -38.6283) -> (138.733, -38.8324)
  line L8309 (139.549, -38.8324) -> (139.549, -38.6283)
  line L8310 (139.549, -38.6283) -> (138.733, -38.6283)
  line L8311 (138.733, -38.8324) -> (139.549, -38.8324)
  line L8312 (141.7209, -39.4104) -> (141.5169, -39.4104)
  line L8313 (141.5169, -38.0504) -> (141.7209, -38.0504)
  line L8314 (141.5169, -39.4104) -> (141.5169, -38.0504)
  line L8315 (141.7209, -38.0504) -> (141.7209, -39.4104)
  line L8316 (141.2109, -38.6284) -> (142.0269, -38.6284)
  line L8317 (141.2109, -38.8324) -> (141.2109, -38.6284)
  line L8318 (142.0269, -38.8324) -> (141.2109, -38.8324)
  line L8319 (142.0269, -38.6284) -> (142.0269, -38.8324)
  line L8320 (139.549, -57.8951) -> (139.549, -57.6911)
  line L8321 (138.733, -57.6911) -> (138.733, -57.8951)
  line L8322 (138.733, -57.8951) -> (139.549, -57.8951)
  line L8323 (139.549, -57.6911) -> (138.733, -57.6911)
  line L8324 (141.7209, -57.1131) -> (141.7209, -58.4731)
  line L8325 (141.5169, -57.1131) -> (141.7209, -57.1131)
  line L8326 (141.7209, -58.4731) -> (141.5169, -58.4731)
  line L8327 (141.5169, -58.4731) -> (141.5169, -57.1131)
  line L8328 (142.0269, -57.8951) -> (141.2109, -57.8951)
  line L8329 (141.2109, -57.6911) -> (142.0269, -57.6911)
  line L8330 (141.2109, -57.8951) -> (141.2109, -57.6911)
  line L8331 (142.0269, -57.6911) -> (142.0269, -57.8951)
  line L8332 (157.7831, -19.7823) -> (158.5991, -19.7823)
  line L8333 (158.5991, -19.7823) -> (158.5991, -19.5783)
  line L8334 (158.5991, -19.5783) -> (157.7831, -19.5783)
  line L8335 (157.7831, -19.5783) -> (157.7831, -19.7823)
  line L8336 (160.5669, -20.3604) -> (160.5669, -19.0003)
  line L8337 (160.7709, -20.3604) -> (160.5669, -20.3604)
  line L8338 (160.5669, -19.0003) -> (160.7709, -19.0003)
  line L8339 (160.7709, -19.0003) -> (160.7709, -20.3604)
  line L8340 (160.2609, -19.7823) -> (160.2609, -19.5783)
  line L8341 (160.2609, -19.5783) -> (161.0769, -19.5783)
  line L8342 (161.0769, -19.7823) -> (160.2609, -19.7823)
  line L8343 (161.0769, -19.5783) -> (161.0769, -19.7823)
  line L8344 (158.5991, -76.7538) -> (157.7831, -76.7538)
  line L8345 (157.7831, -76.9578) -> (158.5991, -76.9578)
  line L8346 (157.7831, -76.7538) -> (157.7831, -76.9578)
  line L8347 (158.5991, -76.9578) -> (158.5991, -76.7538)
  line L8348 (160.7709, -76.1758) -> (160.7709, -77.5359)
  line L8349 (160.5669, -77.5359) -> (160.5669, -76.1758)
  line L8350 (160.5669, -76.1758) -> (160.7709, -76.1758)
  line L8351 (160.7709, -77.5359) -> (160.5669, -77.5359)
  line L8352 (160.2609, -76.9579) -> (160.2609, -76.7538)
  line L8353 (160.2609, -76.7538) -> (161.0769, -76.7538)
  line L8354 (161.0769, -76.7538) -> (161.0769, -76.9579)
  line L8355 (161.0769, -76.9579) -> (160.2609, -76.9579)
  line L8356 (158.5991, -57.8951) -> (158.5991, -57.6911)
  line L8357 (157.7831, -57.8951) -> (158.5991, -57.8951)
  line L8358 (157.7831, -57.6911) -> (157.7831, -57.8951)
  line L8359 (158.5991, -57.6911) -> (157.7831, -57.6911)
  line L8360 (160.5669, -57.1131) -> (160.7709, -57.1131)
  line L8361 (160.7709, -58.4731) -> (160.5669, -58.4731)
  line L8362 (160.7709, -57.1131) -> (160.7709, -58.4731)
  line L8363 (160.5669, -58.4731) -> (160.5669, -57.1131)
  line L8364 (160.2609, -57.6911) -> (161.0769, -57.6911)
  line L8365 (161.0769, -57.8951) -> (160.2609, -57.8951)
  line L8366 (160.2609, -57.8951) -> (160.2609, -57.6911)
  line L8367 (161.0769, -57.6911) -> (161.0769, -57.8951)
  line L8368 (157.7831, -38.8324) -> (158.5991, -38.8324)
  line L8369 (158.5991, -38.8324) -> (158.5991, -38.6283)
  line L8370 (157.7831, -38.6283) -> (157.7831, -38.8324)
  line L8371 (158.5991, -38.6283) -> (157.7831, -38.6283)
  line L8372 (160.5669, -39.4104) -> (160.5669, -38.0504)
  line L8373 (160.7709, -38.0504) -> (160.7709, -39.4104)
  line L8374 (160.7709, -39.4104) -> (160.5669, -39.4104)
  line L8375 (160.5669, -38.0504) -> (160.7709, -38.0504)
  line L8376 (160.2609, -38.8324) -> (160.2609, -38.6284)
  line L8377 (160.2609, -38.6284) -> (161.0769, -38.6284)
  line L8378 (161.0769, -38.8324) -> (160.2609, -38.8324)
  line L8379 (161.0769, -38.6284) -> (161.0769, -38.8324)
  line L8380 (176.8331, -19.5783) -> (176.8331, -19.7823)
  line L8381 (177.6491, -19.7823) -> (177.6491, -19.5783)
  line L8382 (177.6491, -19.5783) -> (176.8331, -19.5783)
  line L8383 (176.8331, -19.7823) -> (177.6491, -19.7823)
  line L8384 (179.617, -19.0003) -> (179.821, -19.0003)
  line L8385 (179.821, -20.3604) -> (179.617, -20.3604)
  line L8386 (179.617, -20.3604) -> (179.617, -19.0003)
  line L8387 (179.821, -19.0003) -> (179.821, -20.3604)
  line L8388 (180.127, -19.7823) -> (179.311, -19.7823)
  line L8389 (179.311, -19.7823) -> (179.311, -19.5783)
  line L8390 (179.311, -19.5783) -> (180.127, -19.5783)
  line L8391 (180.127, -19.5783) -> (180.127, -19.7823)
  line L8392 (176.8331, -76.7538) -> (176.8331, -76.9578)
  line L8393 (177.6491, -76.9578) -> (177.6491, -76.7538)
  line L8394 (177.6491, -76.7538) -> (176.8331, -76.7538)
  line L8395 (176.8331, -76.9578) -> (177.6491, -76.9578)
  line L8396 (179.617, -76.1758) -> (179.821, -76.1758)
  line L8397 (179.821, -77.5359) -> (179.617, -77.5359)
  line L8398 (179.821, -76.1758) -> (179.821, -77.5359)
  line L8399 (179.617, -77.5359) -> (179.617, -76.1758)
  line L8400 (180.127, -76.9579) -> (179.311, -76.9579)
  line L8401 (179.311, -76.7538) -> (180.127, -76.7538)
  line L8402 (180.127, -76.7538) -> (180.127, -76.9579)
  line L8403 (179.311, -76.9579) -> (179.311, -76.7538)
  line L8404 (177.6491, -57.8951) -> (177.6491, -57.6911)
  line L8405 (176.8331, -57.6911) -> (176.8331, -57.8951)
  line L8406 (177.6491, -57.6911) -> (176.8331, -57.6911)
  line L8407 (176.8331, -57.8951) -> (177.6491, -57.8951)
  line L8408 (179.821, -58.4731) -> (179.617, -58.4731)
  line L8409 (179.821, -57.1131) -> (179.821, -58.4731)
  line L8410 (179.617, -57.1131) -> (179.821, -57.1131)
  line L8411 (179.617, -58.4731) -> (179.617, -57.1131)
  line L8412 (180.127, -57.8951) -> (179.311, -57.8951)
  line L8413 (179.311, -57.8951) -> (179.311, -57.6911)
  line L8414 (180.127, -57.6911) -> (180.127, -57.8951)
  line L8415 (179.311, -57.6911) -> (180.127, -57.6911)
  line L8416 (177.6491, -38.6283) -> (176.8331, -38.6283)
  line L8417 (176.8331, -38.8324) -> (177.6491, -38.8324)
  line L8418 (176.8331, -38.6283) -> (176.8331, -38.8324)
  line L8419 (177.6491, -38.8324) -> (177.6491, -38.6283)
  line L8420 (179.821, -39.4104) -> (179.617, -39.4104)
  line L8421 (179.617, -38.0504) -> (179.821, -38.0504)
  line L8422 (179.617, -39.4104) -> (179.617, -38.0504)
  line L8423 (179.821, -38.0504) -> (179.821, -39.4104)
  line L8424 (179.311, -38.6284) -> (180.127, -38.6284)
  line L8425 (180.127, -38.8324) -> (179.311, -38.8324)
  line L8426 (180.127, -38.6284) -> (180.127, -38.8324)
  line L8427 (179.311, -38.8324) -> (179.311, -38.6284)
  line L8428 (101.4489, -76.9578) -> (101.4489, -76.7538)
  line L8429 (100.6329, -76.9578) -> (101.4489, -76.9578)
  line L8430 (100.6329, -76.7538) -> (100.6329, -76.9578)
  line L8431 (101.4489, -76.7538) -> (100.6329, -76.7538)
  line L8432 (103.6208, -76.1758) -> (103.6208, -77.5359)
  line L8433 (103.6208, -77.5359) -> (103.4168, -77.5359)
  line L8434 (103.4168, -77.5359) -> (103.4168, -76.1758)
  line L8435 (103.4168, -76.1758) -> (103.6208, -76.1758)
  line L8436 (103.1108, -76.7538) -> (103.9268, -76.7538)
  line L8437 (103.1108, -76.9579) -> (103.1108, -76.7538)
  line L8438 (103.9268, -76.7538) -> (103.9268, -76.9579)
  line L8439 (103.9268, -76.9579) -> (103.1108, -76.9579)
  line L8440 (100.6329, -57.8951) -> (101.4489, -57.8951)
  line L8441 (101.4489, -57.6911) -> (100.6329, -57.6911)
  line L8442 (101.4489, -57.8951) -> (101.4489, -57.6911)
  line L8443 (100.6329, -57.6911) -> (100.6329, -57.8951)
  line L8444 (103.4168, -57.1131) -> (103.6208, -57.1131)
  line L8445 (103.6208, -58.4731) -> (103.4168, -58.4731)
  line L8446 (103.6208, -57.1131) -> (103.6208, -58.4731)
  line L8447 (103.4168, -58.4731) -> (103.4168, -57.1131)
  line L8448 (103.1108, -57.8951) -> (103.1108, -57.6911)
  line L8449 (103.1108, -57.6911) -> (103.9268, -57.6911)
  line L8450 (103.9268, -57.8951) -> (103.1108, -57.8951)
  line L8451 (103.9268, -57.6911) -> (103.9268, -57.8951)
  line L8452 (100.6329, -19.5783) -> (100.6329, -19.7823)
  line L8453 (101.4489, -19.7823) -> (101.4489, -19.5783)
  line L8454 (101.4489, -19.5783) -> (100.6329, -19.5783)
  line L8455 (100.6329, -19.7823) -> (101.4489, -19.7823)
  line L8456 (103.6208, -19.0003) -> (103.6208, -20.3604)
  line L8457 (103.4168, -20.3604) -> (103.4168, -19.0003)
  line L8458 (103.4168, -19.0003) -> (103.6208, -19.0003)
  line L8459 (103.6208, -20.3604) -> (103.4168, -20.3604)
  line L8460 (103.1108, -19.7823) -> (103.1108, -19.5783)
  line L8461 (103.1108, -19.5783) -> (103.9268, -19.5783)
  line L8462 (103.9268, -19.5783) -> (103.9268, -19.7823)
  line L8463 (103.9268, -19.7823) -> (103.1108, -19.7823)
  line L8464 (100.6329, -38.8324) -> (101.4489, -38.8324)
  line L8465 (101.4489, -38.6283) -> (100.6329, -38.6283)
  line L8466 (100.6329, -38.6283) -> (100.6329, -38.8324)
  line L8467 (101.4489, -38.8324) -> (101.4489, -38.6283)
  line L8468 (103.4168, -38.0504) -> (103.6208, -38.0504)
  line L8469 (103.6208, -38.0504) -> (103.6208, -39.4104)
  line L8470 (103.6208, -39.4104) -> (103.4168, -39.4104)
  line L8471 (103.4168, -39.4104) -> (103.4168, -38.0504)
  line L8472 (103.1108, -38.8324) -> (103.1108, -38.6284)
  line L8473 (103.1108, -38.6284) -> (103.9268, -38.6284)
  line L8474 (103.9268, -38.6284) -> (103.9268, -38.8324)
  line L8475 (103.9268, -38.8324) -> (103.1108, -38.8324)
  line L8476 (119.683, -19.7823) -> (120.499, -19.7823)
  line L8477 (120.499, -19.5783) -> (119.683, -19.5783)
  line L8478 (119.683, -19.5783) -> (119.683, -19.7823)
  line L8479 (120.499, -19.7823) -> (120.499, -19.5783)
  line L8480 (122.6709, -19.0003) -> (122.6709, -20.3604)
  line L8481 (122.4669, -19.0003) -> (122.6709, -19.0003)
  line L8482 (122.6709, -20.3604) -> (122.4669, -20.3604)
  line L8483 (122.4669, -20.3604) -> (122.4669, -19.0003)
  line L8484 (122.9769, -19.7823) -> (122.1609, -19.7823)
  line L8485 (122.9769, -19.5783) -> (122.9769, -19.7823)
  line L8486 (122.1609, -19.7823) -> (122.1609, -19.5783)
  line L8487 (122.1609, -19.5783) -> (122.9769, -19.5783)
  line L8488 (120.499, -57.8951) -> (120.499, -57.6911)
  line L8489 (119.683, -57.6911) -> (119.683, -57.8951)
  line L8490 (119.683, -57.8951) -> (120.499, -57.8951)
  line L8491 (120.499, -57.6911) -> (119.683, -57.6911)
  line L8492 (122.6709, -57.1131) -> (122.6709, -58.4731)
  line L8493 (122.4669, -58.4731) -> (122.4669, -57.1131)
  line L8494 (122.6709, -58.4731) -> (122.4669, -58.4731)
  line L8495 (122.4669, -57.1131) -> (122.6709, -57.1131)
  line L8496 (122.9769, -57.8951) -> (122.1609, -57.8951)
  line L8497 (122.1609, -57.6911) -> (122.9769, -57.6911)
  line L8498 (122.9769, -57.6911) -> (122.9769, -57.8951)
  line L8499 (122.1609, -57.8951) -> (122.1609, -57.6911)
  line L8500 (120.499, -38.6283) -> (119.683, -38.6283)
  line L8501 (120.499, -38.8324) -> (120.499, -38.6283)
  line L8502 (119.683, -38.6283) -> (119.683, -38.8324)
  line L8503 (119.683, -38.8324) -> (120.499, -38.8324)
  line L8504 (122.4669, -39.4104) -> (122.4669, -38.0504)
  line L8505 (122.6709, -38.0504) -> (122.6709, -39.4104)
  line L8506 (122.6709, -39.4104) -> (122.4669, -39.4104)
  line L8507 (122.4669, -38.0504) -> (122.6709, -38.0504)
  line L8508 (122.1609, -38.6284) -> (122.9769, -38.6284)
  line L8509 (122.9769, -38.6284) -> (122.9769, -38.8324)
  line L8510 (122.9769, -38.8324) -> (122.1609, -38.8324)
  line L8511 (122.1609, -38.8324) -> (122.1609, -38.6284)
  line L8512 (120.499, -76.9578) -> (120.499, -76.7538)
  line L8513 (120.499, -76.7538) -> (119.683, -76.7538)
  line L8514 (119.683, -76.7538) -> (119.683, -76.9578)
  line L8515 (119.683, -76.9578) -> (120.499, -76.9578)
  line L8516 (122.4669, -76.1758) -> (122.6709, -76.1758)
  line L8517 (122.6709, -77.5359) -> (122.4669, -77.5359)
  line L8518 (122.6709, -76.1758) -> (122.6709, -77.5359)
  line L8519 (122.4669, -77.5359) -> (122.4669, -76.1758)
  line L8520 (122.1609, -76.9579) -> (122.1609, -76.7538)
  line L8521 (122.1609, -76.7538) -> (122.9769, -76.7538)
  line L8522 (122.9769, -76.9579) -> (122.1609, -76.9579)
  line L8523 (122.9769, -76.7538) -> (122.9769, -76.9579)
  line L8524 (6.1988, -76.9578) -> (6.1988, -76.7538)
  line L8525 (6.1988, -76.7538) -> (5.3828, -76.7538)
  line L8526 (5.3828, -76.7538) -> (5.3828, -76.9578)
  line L8527 (5.3828, -76.9578) -> (6.1988, -76.9578)
  line L8528 (8.1666, -76.1758) -> (8.3706, -76.1758)
  line L8529 (8.1666, -77.5359) -> (8.1666, -76.1758)
  line L8530 (8.3706, -76.1758) -> (8.3706, -77.5359)
  line L8531 (8.3706, -77.5359) -> (8.1666, -77.5359)
  line L8532 (7.8606, -76.9579) -> (7.8606, -76.7538)
  line L8533 (8.6766, -76.9579) -> (7.8606, -76.9579)
  line L8534 (7.8606, -76.7538) -> (8.6766, -76.7538)
  line L8535 (8.6766, -76.7538) -> (8.6766, -76.9579)
  line L8536 (25.2488, -76.7538) -> (24.4328, -76.7538)
  line L8537 (24.4328, -76.7538) -> (24.4328, -76.9578)
  line L8538 (24.4328, -76.9578) -> (25.2488, -76.9578)
  line L8539 (25.2488, -76.9578) -> (25.2488, -76.7538)
  line L8540 (27.2167, -76.1758) -> (27.4207, -76.1758)
  line L8541 (27.2167, -77.5359) -> (27.2167, -76.1758)
  line L8542 (27.4207, -77.5359) -> (27.2167, -77.5359)
  line L8543 (27.4207, -76.1758) -> (27.4207, -77.5359)
  line L8544 (27.7267, -76.9579) -> (26.9107, -76.9579)
  line L8545 (27.7267, -76.7538) -> (27.7267, -76.9579)
  line L8546 (26.9107, -76.7538) -> (27.7267, -76.7538)
  line L8547 (26.9107, -76.9579) -> (26.9107, -76.7538)
  line L8548 (43.4828, -76.7538) -> (43.4828, -76.9578)
  line L8549 (44.2988, -76.9578) -> (44.2988, -76.7538)
  line L8550 (44.2988, -76.7538) -> (43.4828, -76.7538)
  line L8551 (43.4828, -76.9578) -> (44.2988, -76.9578)
  line L8552 (46.4707, -76.1758) -> (46.4707, -77.5359)
  line L8553 (46.2667, -76.1758) -> (46.4707, -76.1758)
  line L8554 (46.2667, -77.5359) -> (46.2667, -76.1758)
  line L8555 (46.4707, -77.5359) -> (46.2667, -77.5359)
  line L8556 (45.9607, -76.9579) -> (45.9607, -76.7538)
  line L8557 (46.7767, -76.7538) -> (46.7767, -76.9579)
  line L8558 (46.7767, -76.9579) -> (45.9607, -76.9579)
  line L8559 (45.9607, -76.7538) -> (46.7767, -76.7538)
  line L8560 (62.5329, -19.5783) -> (62.5329, -19.7823)
  line L8561 (62.5329, -19.7823) -> (63.3489, -19.7823)
  line L8562 (63.3489, -19.5783) -> (62.5329, -19.5783)
  line L8563 (63.3489, -19.7823) -> (63.3489, -19.5783)
  line L8564 (65.5208, -20.3604) -> (65.3167, -20.3604)
  line L8565 (65.3167, -20.3604) -> (65.3167, -19.0003)
  line L8566 (65.3167, -19.0003) -> (65.5208, -19.0003)
  line L8567 (65.5208, -19.0003) -> (65.5208, -20.3604)
  line L8568 (65.0107, -19.5783) -> (65.8267, -19.5783)
  line L8569 (65.8267, -19.5783) -> (65.8267, -19.7823)
  line L8570 (65.8267, -19.7823) -> (65.0107, -19.7823)
  line L8571 (65.0107, -19.7823) -> (65.0107, -19.5783)
  line L8572 (63.3489, -76.7538) -> (62.5329, -76.7538)
  line L8573 (62.5329, -76.7538) -> (62.5329, -76.9578)
  line L8574 (63.3489, -76.9578) -> (63.3489, -76.7538)
  line L8575 (62.5329, -76.9578) -> (63.3489, -76.9578)
  line L8576 (65.5208, -77.5359) -> (65.3167, -77.5359)
  line L8577 (65.5208, -76.1758) -> (65.5208, -77.5359)
  line L8578 (65.3167, -76.1758) -> (65.5208, -76.1758)
  line L8579 (65.3167, -77.5359) -> (65.3167, -76.1758)
  line L8580 (65.8267, -76.9579) -> (65.0107, -76.9579)
  line L8581 (65.0107, -76.9579) -> (65.0107, -76.7538)
  line L8582 (65.0107, -76.7538) -> (65.8267, -76.7538)
  line L8583 (65.8267, -76.7538) -> (65.8267, -76.9579)
  line L8584 (63.3489, -38.8324) -> (63.3489, -38.6283)
  line L8585 (62.5329, -38.6283) -> (62.5329, -38.8324)
  line L8586 (63.3489, -38.6283) -> (62.5329, -38.6283)
  line L8587 (62.5329, -38.8324) -> (63.3489, -38.8324)
  line L8588 (65.5208, -39.4104) -> (65.3167, -39.4104)
  line L8589 (65.3167, -39.4104) -> (65.3167, -38.0504)
  line L8590 (65.3167, -38.0504) -> (65.5208, -38.0504)
  line L8591 (65.5208, -38.0504) -> (65.5208, -39.4104)
  line L8592 (65.8267, -38.6284) -> (65.8267, -38.8324)
  line L8593 (65.0107, -38.6284) -> (65.8267, -38.6284)
  line L8594 (65.8267, -38.8324) -> (65.0107, -38.8324)
  line L8595 (65.0107, -38.8324) -> (65.0107, -38.6284)
  line L8596 (63.3489, -57.6911) -> (62.5329, -57.6911)
  line L8597 (62.5329, -57.8951) -> (63.3489, -57.8951)
  line L8598 (63.3489, -57.8951) -> (63.3489, -57.6911)
  line L8599 (62.5329, -57.6911) -> (62.5329, -57.8951)
  line L8600 (65.3167, -58.4731) -> (65.3167, -57.1131)
  line L8601 (65.5208, -57.1131) -> (65.5208, -58.4731)
  line L8602 (65.5208, -58.4731) -> (65.3167, -58.4731)
  line L8603 (65.3167, -57.1131) -> (65.5208, -57.1131)
  line L8604 (65.0107, -57.6911) -> (65.8267, -57.6911)
  line L8605 (65.0107, -57.8951) -> (65.0107, -57.6911)
  line L8606 (65.8267, -57.6911) -> (65.8267, -57.8951)
  line L8607 (65.8267, -57.8951) -> (65.0107, -57.8951)
  line L8608 (81.5829, -38.8324) -> (82.3989, -38.8324)
  line L8609 (82.3989, -38.6283) -> (81.5829, -38.6283)
  line L8610 (81.5829, -38.6283) -> (81.5829, -38.8324)
  line L8611 (82.3989, -38.8324) -> (82.3989, -38.6283)
  line L8612 (84.5708, -39.4104) -> (84.3668, -39.4104)
  line L8613 (84.5708, -38.0504) -> (84.5708, -39.4104)
  line L8614 (84.3668, -38.0504) -> (84.5708, -38.0504)
  line L8615 (84.3668, -39.4104) -> (84.3668, -38.0504)
  line L8616 (84.0608, -38.8324) -> (84.0608, -38.6284)
  line L8617 (84.0608, -38.6284) -> (84.8768, -38.6284)
  line L8618 (84.8768, -38.6284) -> (84.8768, -38.8324)
  line L8619 (84.8768, -38.8324) -> (84.0608, -38.8324)
  line L8620 (81.5829, -76.7538) -> (81.5829, -76.9578)
  line L8621 (81.5829, -76.9578) -> (82.3989, -76.9578)
  line L8622 (82.3989, -76.7538) -> (81.5829, -76.7538)
  line L8623 (82.3989, -76.9578) -> (82.3989, -76.7538)
  line L8624 (84.3668, -77.5359) -> (84.3668, -76.1758)
  line L8625 (84.5708, -77.5359) -> (84.3668, -77.5359)
  line L8626 (84.3668, -76.1758) -> (84.5708, -76.1758)
  line L8627 (84.5708, -76.1758) -> (84.5708, -77.5359)
  line L8628 (84.0608, -76.9579) -> (84.0608, -76.7538)
  line L8629 (84.0608, -76.7538) -> (84.8768, -76.7538)
  line L8630 (84.8768, -76.9579) -> (84.0608, -76.9579)
  line L8631 (84.8768, -76.7538) -> (84.8768, -76.9579)
  line L8632 (81.5829, -19.7823) -> (82.3989, -19.7823)
  line L8633 (81.5829, -19.5783) -> (81.5829, -19.7823)
  line L8634 (82.3989, -19.7823) -> (82.3989, -19.5783)
  line L8635 (82.3989, -19.5783) -> (81.5829, -19.5783)
  line L8636 (84.3668, -19.0003) -> (84.5708, -19.0003)
  line L8637 (84.5708, -20.3604) -> (84.3668, -20.3604)
  line L8638 (84.5708, -19.0003) -> (84.5708, -20.3604)
  line L8639 (84.3668, -20.3604) -> (84.3668, -19.0003)
  line L8640 (84.0608, -19.7823) -> (84.0608, -19.5783)
  line L8641 (84.0608, -19.5783) -> (84.8768, -19.5783)
  line L8642 (84.8768, -19.7823) -> (84.0608, -19.7823)
  line L8643 (84.8768, -19.5783) -> (84.8768, -19.7823)
  line L8644 (81.5829, -57.8951) -> (82.3989, -57.8951)
  line L8645 (81.5829, -57.6911) -> (81.5829, -57.8951)
  line L8646 (82.3989, -57.6911) -> (81.5829, -57.6911)
  line L8647 (82.3989, -57.8951) -> (82.3989, -57.6911)
  line L8648 (84.3668, -58.4731) -> (84.3668, -57.1131)
  line L8649 (84.5708, -58.4731) -> (84.3668, -58.4731)
  line L8650 (84.5708, -57.1131) -> (84.5708, -58.4731)
  line L8651 (84.3668, -57.1131) -> (84.5708, -57.1131)
  line L8652 (84.0608, -57.6911) -> (84.8768, -57.6911)
  line L8653 (84.8768, -57.8951) -> (84.0608, -57.8951)
  line L8654 (84.0608, -57.8951) -> (84.0608, -57.6911)
  line L8655 (84.8768, -57.6911) -> (84.8768, -57.8951)
  line L8656 (5.3828, -57.8951) -> (6.1988, -57.8951)
  line L8657 (5.3828, -57.6911) -> (5.3828, -57.8951)
  line L8658 (6.1988, -57.8951) -> (6.1988, -57.6911)
  line L8659 (6.1988, -57.6911) -> (5.3828, -57.6911)
  line L8660 (8.1666, -58.4731) -> (8.1666, -57.1131)
  line L8661 (8.3706, -57.1131) -> (8.3706, -58.4731)
  line L8662 (8.1666, -57.1131) -> (8.3706, -57.1131)
  line L8663 (8.3706, -58.4731) -> (8.1666, -58.4731)
  line L8664 (7.8606, -57.8951) -> (7.8606, -57.6911)
  line L8665 (7.8606, -57.6911) -> (8.6766, -57.6911)
  line L8666 (8.6766, -57.6911) -> (8.6766, -57.8951)
  line L8667 (8.6766, -57.8951) -> (7.8606, -57.8951)
  line L8668 (5.3828, -19.7823) -> (6.1988, -19.7823)
  line L8669 (6.1988, -19.5783) -> (5.3828, -19.5783)
  line L8670 (6.1988, -19.7823) -> (6.1988, -19.5783)
  line L8671 (5.3828, -19.5783) -> (5.3828, -19.7823)
  line L8672 (8.1666, -20.3604) -> (8.1666, -19.0003)
  line L8673 (8.3706, -20.3604) -> (8.1666, -20.3604)
  line L8674 (8.3706, -19.0003) -> (8.3706, -20.3604)
  line L8675 (8.1666, -19.0003) -> (8.3706, -19.0003)
  line L8676 (8.6766, -19.7823) -> (7.8606, -19.7823)
  line L8677 (7.8606, -19.7823) -> (7.8606, -19.5783)
  line L8678 (7.8606, -19.5783) -> (8.6766, -19.5783)
  line L8679 (8.6766, -19.5783) -> (8.6766, -19.7823)
  line L8680 (6.1988, -38.8324) -> (6.1988, -38.6283)
  line L8681 (5.3828, -38.8324) -> (6.1988, -38.8324)
  line L8682 (5.3828, -38.6283) -> (5.3828, -38.8324)
  line L8683 (6.1988, -38.6283) -> (5.3828, -38.6283)
  line L8684 (8.1666, -38.0504) -> (8.3706, -38.0504)
  line L8685 (8.3706, -39.4104) -> (8.1666, -39.4104)
  line L8686 (8.3706, -38.0504) -> (8.3706, -39.4104)
  line L8687 (8.1666, -39.4104) -> (8.1666, -38.0504)
  line L8688 (8.6766, -38.8324) -> (7.8606, -38.8324)
  line L8689 (8.6766, -38.6284) -> (8.6766, -38.8324)